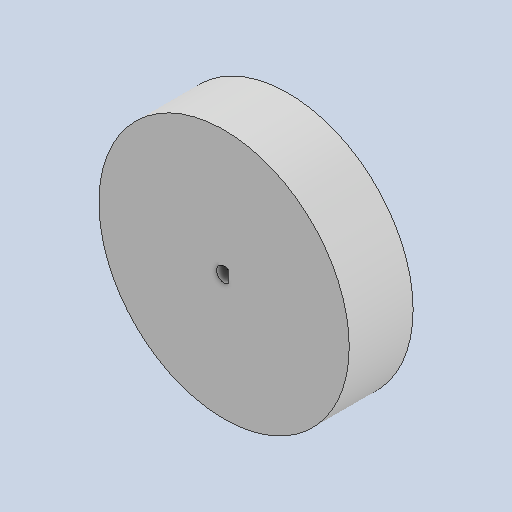
# Autodesk Inventor part: Wheel
Saved by Autodesk Inventor 2023 (Build 270158000, 158)
## iProperties
Created: 2023-10-05
Part Number: Wheel
Material: Generic
Document SubType Name: Modeling
Designer: say514
Density: 1 g/cm^3
Appearance: Default
Author: say514
Autodesk Inventor part; units mm, degrees
ref_plane "YZ Plane" through (0, 0, 0) normal (1, 0, 0) x (0, 1, 0)
ref_plane "XZ Plane" through (0, 0, 0) normal (0, 1, 0) x (-1, 0, 0)
ref_plane "XY Plane" through (0, 0, 0) normal (0, 0, 1) x (1, 0, 0)
ref_plane "Work Plane2" through (0, 0, 0) normal (0, 0, 1) x (1, 0, 0)
sketch "Wheel Sketch" plane through (0, 0, 0) normal (0, 0, 1) x (1, 0, 0)
  circle A0 centre (0, 0) radius 23.5
  dimension "d0" = 47
  constraints: 1 centre point
  measures "d0" diameter of A0
extrude "Extrusion1" add sketch "Wheel Sketch" along normal blind 12
sketch "Sketch2" plane through (0, 0, 0) normal (0, 0, 1) x (1, 0, 0)
  arc A0 (0.8, 1.1489) -> (0.8, -1.1489) centre (0, 0) ccw
  line L0 (0.8, 0) -> (0.8, 1.1489)
  line L1 (0.8, 0) -> (0.8, -1.1489)
  constraints: 4 end point, 2 point on circle, 1 centre point, 1 coincident, 1 vertical
extrude "Extrusion2" cut sketch "Sketch2" along normal blind 12
body "Solid1"
